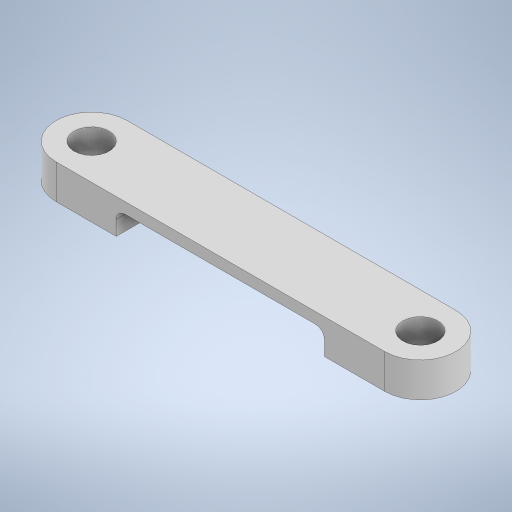
# Autodesk Inventor part: dol_trzymacz
Saved by Autodesk Inventor 2023 (Build 270158000, 158)
## iProperties
Created: 2024-05-17
Part Number: dol_trzymacz
Material: Ogólny
Document SubType Name: Modeling
Designer: kamil
Density: 1 g/cm^3
Appearance: Domyślna
Author: kamil
Autodesk Inventor part; units mm, degrees
ref_plane "YZ Plane" through (0, 0, 0) normal (1, 0, 0) x (0, 1, 0)
ref_plane "XZ Plane" through (0, 0, 0) normal (0, 1, 0) x (-1, 0, 0)
ref_plane "XY Plane" through (0, 0, 0) normal (0, 0, 1) x (1, 0, 0)
sketch "Szkic1" plane through (0, 0, 0) normal (0, 1, 0) x (-1, 0, 0)
  line L0 (9.5668, 14.1781) -> (9.5668, 20.6781)
  line L1 (15.0668, 14.1781) -> (9.5668, 14.1781)
  arc A0 (15.0668, 14.1781) -> (15.0668, 20.6781) centre (15.0668, 17.4281) ccw
  line L2 (9.5668, 20.6781) -> (15.0668, 20.6781)
  circle A1 centre (15.0668, 17.4281) radius 1.6
  line L3 (-14.9332, 20.6781) -> (-9.4332, 20.6781)
  arc A2 (-14.9332, 20.6781) -> (-14.9332, 14.1781) centre (-14.9332, 17.4281) ccw
  line L4 (-9.4332, 14.1781) -> (-14.9332, 14.1781)
  line L5 (-9.4332, 20.6781) -> (-9.4332, 14.1781)
  circle A3 centre (-14.9332, 17.4281) radius 1.6
  point P0 (0, 0)
  constraints: 12 end point, 4 centre point, 4 point on circle
extrude "Wyciągnięcie proste1" add sketch "Szkic1" along normal blind 3.15
sketch "Szkic2" plane through (0, 3.15, 0) normal (0, 1, 0) x (1, 0, 0)
  line L0 (-9.5668, -20.6781) -> (-9.5668, -14.1781) projected
  line L1 (9.4332, -14.1781) -> (9.4332, -20.6781) projected
  line L2 (-15.0668, -20.6781) -> (-9.5668, -20.6781) projected
  line L3 (9.4332, -14.1781) -> (9.4332, -20.6781) projected
  line L4 (-9.5668, -20.6781) -> (9.4332, -20.6781)
  line L5 (-9.5668, -14.1781) -> (-15.0668, -14.1781) projected
  line L6 (9.4332, -14.1781) -> (-9.5668, -14.1781)
  point P0 (0, 0)
  constraints: 4 end point, 1 collinear, 1 perpendicular
extrude "Wyciągnięcie proste2" add sketch "Szkic2" against normal blind 1
fillet "Zaokrąglenie1" radius 0.8 2 edges at (9.4332, 2.15, 17.4281) (-9.5668, 2.15, 17.4281)
